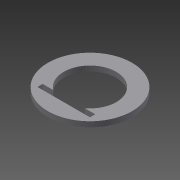
# Autodesk Inventor part: Part1
Saved by Autodesk Inventor 2014 SP1 (Build 180222100, 222)
## iProperties
Created: 2018-05-14
Part Number: Part1
Material: Generic
Document SubType Name: Modeling
Designer: Dadang
Density: 1 g/cm^3
Appearance: Default
Author: Dadang
Autodesk Inventor part; units mm, degrees
ref_plane "YZ Plane" through (0, 0, 0) normal (1, 0, 0) x (0, 1, 0)
ref_plane "XZ Plane" through (0, 0, 0) normal (0, 1, 0) x (-1, 0, 0)
ref_plane "XY Plane" through (0, 0, 0) normal (0, 0, 1) x (1, 0, 0)
sketch "Sketch1" plane through (0, 0, 0) normal (0, 0, 1) x (1, 0, 0)
  circle A0 centre (0, 0) radius 40
  arc A1 (15, -20) -> (-15, -20) centre (0, 0) ccw
  line L0 (0, -25) -> (-25, -25)
  line L1 (-25, -25) -> (-25, -20)
  line L2 (25, -20) -> (25, -25)
  line L3 (25, -25) -> (0, -25)
  line L4 (-25, -20) -> (-15, -20)
  line L5 (15, -20) -> (25, -20)
  dimension "d0" = 80
  dimension "d1" = 50
  dimension "d2" = 25
  dimension "d3" = 5
  dimension "d4" = 50
  constraints: 12 end point, 4 parallel, 3 perpendicular, 2 centre point, 2 coincident, 2 point on circle, 2 tangent, 1 horizontal
  measures "d0" diameter of A0
  measures "d1" diameter of A1
  measures "d2" distance of L0.start L0.end
  measures "d3" distance of L0.end L1.end
  measures "d4" distance of L1.end L2.start
extrude "Extrusion1" add sketch "Sketch1" along normal blind 5
body "Solid1"
